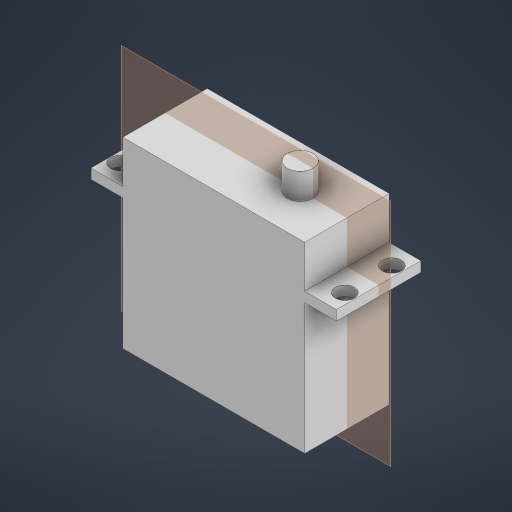
# Autodesk Inventor part: 40kgServo
Saved by Autodesk Inventor 2024 (Build 280153000, 153)
## iProperties
Created: 2025-10-08
Part Number: 40kgServo
Material: Generic
Document SubType Name: Modeling
Designer: kevin
Density: 1 g/cm^3
Appearance: Default
Author: kevin
Autodesk Inventor part; units mm, degrees
ref_plane "YZ Plane" through (0, 0, 0) normal (1, 0, 0) x (0, 1, 0)
ref_plane "XZ Plane" through (0, 0, 0) normal (0, 1, 0) x (-1, 0, 0)
ref_plane "XY Plane" through (0, 0, 0) normal (0, 0, 1) x (1, 0, 0)
sketch "Sketch2" plane through (0, 0, 0) normal (0, 0, 1) x (1, 0, 0)
  line L0 (-20.195, -14.5) -> (20.195, -14.5)
  line L1 (20.195, -14.5) -> (20.195, 14.5)
  line L2 (20.195, 14.5) -> (-20.195, 14.5)
  line L3 (-20.195, 14.5) -> (-20.195, -14.5)
  line L4 (-20.195, -14.5) -> (20.195, 14.5) construction
  line L5 (20.195, -14.5) -> (-20.195, 14.5) construction
  point P0 (0, 0)
  dimension "d0" = 40.39
  dimension "d1" = 29
  constraints: 12 end point, 2 midpoint, 2 parallel, 1 horizontal, 1 perpendicular
  measures "d0" distance of L2.end L1.end
  measures "d1" distance of L1.end L0.end
extrude "Extrusion1" add sketch "Sketch2" along normal blind 18.75
sketch "Sketch3" plane through (-20.195, 14.5, 0) normal (0, 1, 0) x (1, 0, 0)
  line L0 (40.39, 0) -> (0, 0) construction
  line L1 (0, 0) -> (0, -18.75) construction
  line L2 (40.39, -18.75) -> (0, -18.75) construction
  line L3 (40.39, 0) -> (40.39, -18.75) construction
  line L4 (0, 0) -> (40.39, -18.75) construction
  line L5 (-7.045, -18.75) -> (47.435, -18.75)
  line L6 (47.435, -18.75) -> (47.435, 0)
  line L7 (47.435, 0) -> (-7.045, 0)
  line L8 (-7.045, 0) -> (-7.045, -18.75)
  line L9 (-7.045, -18.75) -> (47.435, 0) construction
  line L10 (47.435, -18.75) -> (-7.045, 0) construction
  line L11 (-7.045, -9.375) -> (47.435, -9.375) construction
  circle A0 centre (-4.75, -4.15) radius 2.1
  line L12 (20.195, -9.375) -> (20.195, -3.4775) construction
  circle A1 centre (-4.75, -14.6) radius 2.1
  circle A2 centre (45.14, -4.15) radius 2.1
  circle A3 centre (45.14, -14.6) radius 2.1
  point P0 (20.195, 0)
  dimension "d4" = 54.48
  dimension "d5" = 4.2
  dimension "d6" = 4.15
  dimension "d7" = 4.75
  constraints: 18 end point, 5 midpoint, 4 centre point, 3 symmetric about line, 2 parallel, 1 horizontal, 1 perpendicular, 1 vertical, 3 other
  measures "d4" distance of L7.end L6.end
  measures "d5" diameter of A0
  measures "d6" distance from line of L7 A0.centre
  measures "d7" distance from line of A0.centre L1
extrude "Extrusion2" add sketch "Sketch3" along normal blind 2.22
sketch "Sketch4" plane through (-20.195, 16.72, 0) normal (0, 1, 0) x (1, 0, 0)
  line L0 (0, 0) -> (0, -18.75) projected
  line L1 (40.39, 0) -> (40.39, -18.75) projected
  line L2 (47.435, 0) -> (-7.045, 0) projected
  line L3 (-7.045, -18.75) -> (47.435, -18.75) projected
  point P0 (20.195, 0)
extrude "Extrusion3" add sketch "Sketch4" along normal blind 9.42
sketch "Sketch5" plane through (-20.195, 26.14, 0) normal (0, 1, 0) x (1, 0, 0)
  line L0 (40.39, -18.75) -> (40.39, 0) projected
  line L1 (40.39, 0) -> (0, 0) projected
  line L2 (0, 0) -> (0, -18.75) projected
  line L3 (0, -18.75) -> (40.39, -18.75) projected
  line L4 (40.39, -9.375) -> (0, -9.375) construction
  circle A0 centre (30, -9.375) radius 2.865
  point P0 (20.195, 0)
  dimension "d12" = 30
  dimension "d13" = 5.73
  constraints: 2 end point, 2 midpoint, 1 centre point, 1 point on line
  measures "d12" distance from line of L2 A0.centre
  measures "d13" diameter of A0
extrude "Extrusion4" add sketch "Sketch5" along normal blind 5.77 contours A0
ref_plane "Work Plane1" through (0, 0, 9.375) normal (0, 0, 1) x (1, 0, 0)
body "Solid1"
